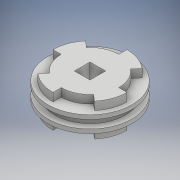
# Autodesk Inventor part: dog clutch
Saved by Autodesk Inventor 2017 (Build 210142000, 142)
## iProperties
Created: 2018-04-16
Part Number: dog clutch
Material: Generic
Document SubType Name: Modeling
Designer: RKL
Density: 1 g/cm^3
Appearance: Default
Author: RKL
Autodesk Inventor part; units mm, degrees
ref_plane "YZ Plane" through (0, 0, 0) normal (1, 0, 0) x (0, 1, 0)
ref_plane "XZ Plane" through (0, 0, 0) normal (0, 1, 0) x (-1, 0, 0)
sketch "Sketch1" plane through (0, 0, 0) normal (0, 0, 1) x (1, 0, 0)
  circle A0 centre (0, 0) radius 17.5
  circle A1 centre (0, 0) radius 25.5
  dimension "d0" = 35
  dimension "d1" = 8
  constraints: 2 centre point, 2 coincident
  measures "d0" diameter of A0
  measures "d1" radial gap between concentric circles of A0 A1
extrude "Extrusion1" add sketch "Sketch1" along normal blind 10
ref_plane "Work Plane1" through (0, 0, 5) normal (0, 0, 1) x (1, 0, 0)
sketch "Sketch2" plane through (0, 0, 5) normal (0, 0, 1) x (1, 0, 0)
  circle A0 centre (0, 0) radius 25.5 projected
  circle A1 centre (0, 0) radius 21.5
  dimension "d4" = 4
  constraints: 1 centre point, 1 coincident
  measures "d4" radial gap between concentric circles of A0 A1
extrude "Extrusion2" cut sketch "Sketch2" along normal mid plane 5
sketch "Sketch3" plane through (0, 0, 10) normal (0, 0, 1) x (1, 0, 0)
  circle A0 centre (0, 0) radius 17.5 construction
  line L0 (0, 0) -> (0, 17.5) construction
  line L1 (0, 17.5) -> (0, 22.5)
  arc A1 (14.4627, 17.236) -> (0, 22.5) centre (0, 0) ccw
  arc A2 (11.2488, 13.4058) -> (0, 17.5) centre (0, 0) ccw
  line L2 (14.4627, 17.236) -> (11.2488, 13.4058)
  dimension "d7" = 5
  dimension "d8" = 40
  constraints: 6 end point, 4 point on circle, 2 centre point, 2 coincident, 1 line through centre, 1 point on line, 1 vertical, 1 vertical alignment, 1 other
  measures "d7" distance of L0.end L1.end
  measures "d8" angle of L1 L2
extrude "Extrusion3" add sketch "Sketch3" along normal blind 5
pattern_circular "Circular Pattern1" count 4 over 360 about axis through (0, 0, 0) along (0, 0, 1) of "Extrusion3"
mirror "Mirror1" about plane through (0, 0, 5) normal (0, 0, 1) of "Extrusion3", "Circular Pattern1"
sketch "Sketch4" plane through (0, 0, 10) normal (0, 0, 1) x (1, 0, 0)
  arc A0 (17.5, 0) -> (11.2488, 13.4058) centre (0, 0) ccw projected
  arc A1 (11.2488, 13.4058) -> (0, 17.5) centre (0, 0) ccw projected
  arc A2 (0, 17.5) -> (-13.4058, 11.2488) centre (0, 0) ccw projected
  arc A3 (-13.4058, 11.2488) -> (-17.5, 0) centre (0, 0) ccw projected
  arc A4 (-17.5, 0) -> (-11.2488, -13.4058) centre (0, 0) ccw projected
  arc A5 (-11.2488, -13.4058) -> (0, -17.5) centre (0, 0) ccw projected
  arc A6 (0, -17.5) -> (13.4058, -11.2488) centre (0, 0) ccw projected
  arc A7 (13.4058, -11.2488) -> (17.5, 0) centre (0, 0) ccw projected
  line L0 (4.7625, -4.7625) -> (-4.7625, -4.7625)
  line L1 (-4.7625, -4.7625) -> (-4.7625, 4.7625)
  line L2 (-4.7625, 4.7625) -> (4.7625, 4.7625)
  line L3 (4.7625, 4.7625) -> (4.7625, -4.7625)
  line L4 (4.7625, -4.7625) -> (-4.7625, 4.7625) construction
  line L5 (-4.7625, -4.7625) -> (4.7625, 4.7625) construction
  arc A8 (0, 17.5) -> (-13.4058, 11.2488) centre (0, 0) ccw projected
  circle A9 centre (0, 0) radius 17.5
  dimension "d14" = 9.525
  constraints: 12 end point, 2 midpoint, 2 parallel, 2 perpendicular, 1 coincident, 1 horizontal, 3 other
  measures "d14" distance of L0.end L1.end
extrude "Extrusion4" add sketch "Sketch4" against normal up to surface (20 mm away) from surface at 5
body "Solid1"
